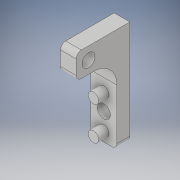
# Autodesk Inventor part: BR
Saved by Autodesk Inventor 2019 (Build 230136000, 136)
## iProperties
Created: 2020-07-09
Part Number: BR
Material: Generic
Document SubType Name: Modeling
Designer: infinity
Density: 1 g/cm^3
Appearance: Default
Author: infinity
Autodesk Inventor part; units mm, degrees
ref_plane "YZ Plane" through (0, 0, 0) normal (1, 0, 0) x (0, 1, 0)
ref_plane "XZ Plane" through (0, 0, 0) normal (0, 1, 0) x (-1, 0, 0)
ref_plane "XY Plane" through (0, 0, 0) normal (0, 0, 1) x (1, 0, 0)
sketch "Sketch1" plane through (0, 0, 0) normal (1, 0, 0) x (0, 1, 0)
  line L0 (0, 0) -> (15.25, 0)
  line L1 (15.25, 0) -> (15.25, 7.825)
  line L2 (15.25, 7.825) -> (20, 7.825)
  line L3 (20, 7.825) -> (20, -2.5)
  line L4 (20, -2.5) -> (0, -2.5)
  line L5 (0, -2.5) -> (0, 0)
  point P0 (17.625, 5.45)
  dimension "d8" = 2.5
  dimension "d21" = 5.45
  dimension "d23" = 20
  dimension "d24" = 2.375
  dimension "d25" = 2.375
  dimension "d26" = 2.375
  constraints: 12 end point, 5 perpendicular, 1 horizontal
  measures "d8" distance between parallel lines of L4 L0
  measures "d21" distance from line of L0 point (17.625, 5.45)
  measures "d23" distance between parallel lines of L3 L5
  measures "d24" distance from line of L3 point (17.625, 5.45)
  measures "d25" distance from line of L1 point (17.625, 5.45)
  measures "d26" distance from line of point (17.625, 5.45) L2
extrude "Extrusion1" add sketch "Sketch1" along normal blind 5
sketch "Sketch2" plane through (0, 0, 0) normal (0, 0, 1) x (1, 0, 0)
  line L0 (2.5, 1.9) -> (2.5, 8.35) construction
  line L1 (5, 15.25) -> (5, 0) construction
  line L2 (0, 0) -> (0, 15.25) construction
  circle A0 centre (2.5, 8.35) radius 1
  circle A1 centre (2.5, 1.9) radius 1
  line L3 (0, 0) -> (5, 0) projected
  line L4 (0, 15.25) -> (5, 15.25) projected
  point P0 (2.5, 5.125)
  dimension "d2" = 5
  dimension "d3" = 2.5
  dimension "d4" = 8.45
  dimension "d5" = 2
  dimension "d6" = 2
  dimension "d27" = 5.125
  constraints: 4 coincident, 2 centre point, 2 end point, 1 midpoint, 1 vertical
  measures "d2" distance between parallel lines of L1 L2
  measures "d3" distance between parallel lines of L0 L2
  measures "d5" diameter of A0
  measures "d6" diameter of A1
  measures "d27" distance from line of L3 point (2.5, 5.125)
extrude "Extrusion2" add sketch "Sketch2" along normal blind 2
hole "Hole1" at (2.5, 5.125, 0) direction (0, 0, -1) diameter 2.53 end through all
fillet "Fillet1" radius 1 2 edges at (5, 0, -1.25) (0, 0, -1.25)
sketch "Sketch3" plane through (5, 20, -2.5) normal (0, 0, -1) x (-1, 0, 0)
  line L0 (5, 0) -> (5, -19) projected
  line L1 (5, 0) -> (3, 0)
  line L2 (3, 0) -> (3, -7.5)
  line L3 (3, -7.5) -> (5, -7.5)
  line L4 (5, -7.5) -> (5, 0)
  line L5 (0, -19) -> (0, 0) projected
  point P0 (5, -20)
  dimension "d28" = 3
  dimension "d29" = 7.5
  constraints: 8 end point, 2 parallel, 1 horizontal, 1 perpendicular
  measures "d28" distance between parallel lines of L5 L2
  measures "d29" distance between parallel lines of L1 L3
extrude "Extrusion3" cut sketch "Sketch3" against normal up to surface (10.325 mm away)
hole "Hole2" at (0, 17.625, 5.45) direction (1, 0, 0) diameter 2.5 end through all
fillet "Fillet2" radius 1 4 edges at (0, 12.5, -1.25) (2, 12.5, -1.25) (3.5, 15.25, 7.825) (3.5, 20, 7.825)
fillet "Fillet2" radius 4.5 1 edges at (3.5, 15.25, 0)
equation "\"d26\" = d24"
equation "\"d3\" = 0.5 * d2"
equation "\"d6\" = d5"
body "Solid1"
